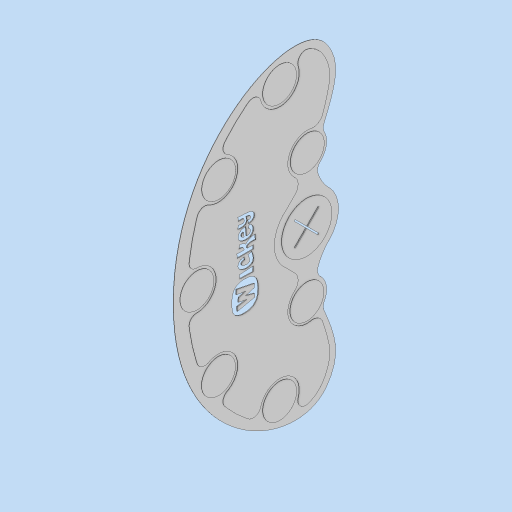
# Autodesk Inventor part: Sticker5
Saved by Autodesk Inventor 2024 (Build 280153000, 153)
## iProperties
Created: 2025-01-25
Part Number: Sticker5
Material: Generic
Document SubType Name: Modeling
Designer: Dmitry
Density: 1 g/cm^3
Appearance: Default
Author: Dmitry
Autodesk Inventor part; units mm, degrees
(part 1 of 2)
ref_plane "YZ Plane" through (0, 0, 0) normal (1, 0, 0) x (0, 1, 0)
ref_plane "XZ Plane" through (0, 0, 0) normal (0, 1, 0) x (-1, 0, 0)
ref_plane "XY Plane" through (0, 0, 0) normal (0, 0, 1) x (1, 0, 0)
sketch "Sketch1" plane through (0, 0, 0) normal (1, 0, 0) x (0, 1, 0)
  line L0 (189.6656, 2.8121) -> (188.0501, 2.8121)
  line L1 (188.0501, 2.8121) -> (183.2013, 3.4446)
  line L2 (183.2013, 3.4446) -> (176.455, 5.1464)
  line L3 (176.455, 5.1464) -> (169.3456, 7.6325)
  line L4 (169.3456, 7.6325) -> (163.6712, 9.8611)
  line L5 (163.6712, 9.8611) -> (161.7865, 10.6188)
  line L6 (161.7865, 10.6188) -> (160.3946, 11.1784)
  line L7 (160.3946, 11.1784) -> (156.2163, 12.8403)
  line L8 (137.2895, 19.2866) -> (130.161, 21.0285)
  line L9 (130.161, 21.0285) -> (122.5829, 22.3971)
  line L10 (108.1191, 23.6122) -> (105.9832, 23.6122)
  line L11 (105.9832, 23.6122) -> (105.6538, 23.6122)
  line L12 (103.6515, 23.6122) -> (103.3513, 23.6122)
  line L13 (103.3513, 23.6122) -> (101.2136, 23.6122)
  line L14 (86.7498, 22.3971) -> (79.1723, 21.0285)
  line L15 (79.1723, 21.0285) -> (72.0448, 19.2866)
  line L16 (48.9404, 11.1784) -> (47.5516, 10.6188)
  line L17 (47.5516, 10.6188) -> (45.6651, 9.8611)
  line L18 (45.6651, 9.8611) -> (39.9902, 7.6325)
  line L19 (39.9902, 7.6325) -> (32.8782, 5.1451)
  line L20 (32.8782, 5.1451) -> (26.1327, 3.4433)
  line L21 (26.1327, 3.4433) -> (21.2849, 2.8121)
  line L22 (21.2849, 2.8121) -> (19.67, 2.8121)
  line L23 (19.67, 2.8121) -> (18.5219, 2.8121)
  line L24 (18.5219, 2.8121) -> (15.0822, 3.1842)
  line L25 (15.0822, 3.1842) -> (10.6893, 4.3171)
  line L26 (10.6893, 4.3171) -> (6.4089, 6.2381)
  line L27 (6.4089, 6.2381) -> (3.179, 8.2239)
  line L28 (3.179, 8.2239) -> (2.1686, 8.9734)
  line L29 (2.1686, 8.9734) -> (1.3914, 9.551)
  line L30 (1.3914, 9.551) -> (-0.6922, 11.6137)
  line L31 (-0.6922, 11.6137) -> (-2.9411, 14.8096)
  line L32 (-2.9411, 14.8096) -> (-4.5728, 18.5121)
  line L33 (-4.5728, 18.5121) -> (-5.5802, 22.6739)
  line L34 (-5.5802, 22.6739) -> (-5.9535, 27.2477)
  line L35 (-5.9535, 27.2477) -> (-5.6861, 32.1824)
  line L36 (-5.6861, 32.1824) -> (-4.7712, 37.4326)
  line L37 (-4.7712, 37.4326) -> (-3.6589, 41.588)
  line L38 (-3.6589, 41.588) -> (-3.2004, 42.9444)
  line L39 (-3.2004, 42.9444) -> (-2.6889, 44.4633)
  line L40 (-2.6889, 44.4633) -> (-0.8492, 48.9159)
  line L41 (-0.8492, 48.9159) -> (2.1343, 54.8164)
  line L42 (2.1343, 54.8164) -> (5.7129, 60.5999)
  line L43 (5.7129, 60.5999) -> (9.8498, 66.221)
  line L44 (9.8498, 66.221) -> (14.5062, 71.6312)
  line L45 (14.5062, 71.6312) -> (19.6433, 76.7823)
  line L46 (19.6433, 76.7823) -> (25.2262, 81.6261)
  line L47 (25.2262, 81.6261) -> (29.6814, 85.05)
  line L48 (29.6814, 85.05) -> (31.2163, 86.1168)
  line L49 (31.2163, 86.1168) -> (33.089, 87.4198)
  line L50 (33.089, 87.4198) -> (38.929, 91.019)
  line L51 (38.929, 91.019) -> (47.0789, 95.2938)
  line L52 (47.0789, 95.2938) -> (55.631, 98.9387)
  line L53 (55.631, 98.9387) -> (64.5566, 101.9435)
  line L54 (64.5566, 101.9435) -> (73.8238, 104.2956)
  line L55 (73.8238, 104.2956) -> (83.3986, 105.9872)
  line L56 (83.3986, 105.9872) -> (93.2515, 107.0083)
  line L57 (93.2515, 107.0083) -> (100.825, 107.3512)
  line L58 (100.825, 107.3512) -> (103.3513, 107.3512)
  line L59 (103.3513, 107.3512) -> (103.6007, 107.3512)
  line L60 (103.6007, 107.3512) -> (104.2647, 107.3461)
  line L61 (104.2647, 107.3461) -> (104.3487, 107.3436)
  line L62 (104.3487, 107.3436) -> (104.6894, 107.341)
  line L63 (104.6894, 107.341) -> (104.9853, 107.3436)
  line L64 (104.9853, 107.3436) -> (105.0681, 107.3461)
  line L65 (105.0681, 107.3461) -> (105.7544, 107.3512)
  line L66 (105.7544, 107.3512) -> (105.9832, 107.3512)
  line L67 (105.9832, 107.3512) -> (108.5077, 107.3512)
  line L68 (108.5077, 107.3512) -> (116.0815, 107.0083)
  line L69 (116.0815, 107.0083) -> (125.9342, 105.9872)
  line L70 (125.9342, 105.9872) -> (135.509, 104.2956)
  line L71 (135.509, 104.2956) -> (144.7761, 101.9435)
  line L72 (144.7761, 101.9435) -> (153.7017, 98.9387)
  line L73 (153.7017, 98.9387) -> (162.2564, 95.2938)
  line L74 (162.2564, 95.2938) -> (170.4047, 91.019)
  line L75 (170.4047, 91.019) -> (176.2442, 87.4198)
  line L76 (176.2442, 87.4198) -> (178.1187, 86.1168)
  line L77 (178.1187, 86.1168) -> (179.6554, 85.05)
  line L78 (179.6554, 85.05) -> (184.108, 81.6261)
  line L79 (184.108, 81.6261) -> (189.691, 76.7823)
  line L80 (189.691, 76.7823) -> (194.8268, 71.6312)
  line L81 (194.8268, 71.6312) -> (199.4852, 66.221)
  line L82 (199.4852, 66.221) -> (203.6203, 60.5999)
  line L83 (203.6203, 60.5999) -> (207.1992, 54.8164)
  line L84 (207.1992, 54.8164) -> (210.1837, 48.9159)
  line L85 (210.1837, 48.9159) -> (212.0226, 44.4633)
  line L86 (212.0226, 44.4633) -> (212.5357, 42.9444)
  line L87 (212.5357, 42.9444) -> (212.9929, 41.588)
  line L88 (212.9929, 41.588) -> (214.1029, 37.4326)
  line L89 (214.1029, 37.4326) -> (215.0198, 32.1824)
  line L90 (215.0198, 32.1824) -> (215.2865, 27.2477)
  line L91 (215.2865, 27.2477) -> (214.9132, 22.6739)
  line L92 (214.9132, 22.6739) -> (213.9073, 18.5121)
  line L93 (213.9073, 18.5121) -> (212.2741, 14.8096)
  line L94 (212.2741, 14.8096) -> (210.0237, 11.6137)
  line L95 (210.0237, 11.6137) -> (207.9434, 9.5495)
  line L96 (207.9434, 9.5495) -> (207.1662, 8.9734)
  line L97 (207.1662, 8.9734) -> (206.1552, 8.2239)
  line L98 (206.1552, 8.2239) -> (202.9244, 6.2381)
  line L99 (202.9244, 6.2381) -> (198.647, 4.3171)
  line L100 (198.647, 4.3171) -> (194.2528, 3.1842)
  line L101 (194.2528, 3.1842) -> (190.8136, 2.8121)
  line L102 (190.8136, 2.8121) -> (189.6681, 2.8121)
  line L103 (189.6681, 2.8121) -> (189.6656, 2.8121)
  line L104 (205.0808, 10.3404) -> (204.0877, 9.6277)
  line L105 (204.0877, 9.6277) -> (200.9254, 7.7481)
  line L106 (200.9254, 7.7481) -> (196.7318, 5.928)
  line L107 (196.7318, 5.928) -> (192.4265, 4.8543)
  line L108 (192.4265, 4.8543) -> (189.0585, 4.5017)
  line L109 (189.0585, 4.5017) -> (187.9358, 4.5017)
  line L110 (187.9358, 4.5017) -> (186.8157, 4.5017)
  line L111 (186.8157, 4.5017) -> (183.4603, 4.9744)
  line L112 (183.4603, 4.9744) -> (178.0984, 6.1774)
  line L113 (178.0984, 6.1774) -> (172.4977, 7.7895)
  line L114 (172.4977, 7.7895) -> (168.5937, 9.045)
  line L115 (168.5937, 9.045) -> (167.3034, 9.4875)
  line L116 (167.3034, 9.4875) -> (166.7192, 9.6872)
  line L117 (166.7192, 9.6872) -> (165.1165, 10.7098)
  line L118 (165.1165, 10.7098) -> (163.5391, 12.5632)
  line L119 (163.5391, 12.5632) -> (162.7009, 14.8398)
  line L120 (162.7009, 14.8398) -> (162.6196, 16.7318)
  line L121 (162.6196, 16.7318) -> (162.7466, 17.3298)
  line L122 (162.7466, 17.3298) -> (162.8127, 17.6577)
  line L123 (162.8127, 17.6577) -> (163.0108, 19.3392)
  line L124 (163.0108, 19.3392) -> (163.0057, 21.074)
  line L125 (163.0057, 21.074) -> (162.9752, 21.4268)
  line L126 (162.9752, 21.4268) -> (162.9194, 22.0262)
  line L127 (162.9194, 22.0262) -> (162.5358, 23.804)
  line L128 (162.5358, 23.804) -> (161.7002, 26.0196)
  line L129 (161.7002, 26.0196) -> (160.5089, 28.0359)
  line L130 (160.5089, 28.0359) -> (159.0001, 29.8134)
  line L131 (159.0001, 29.8134) -> (157.2145, 31.3114)
  line L132 (157.2145, 31.3114) -> (155.1927, 32.4925)
  line L133 (155.1927, 32.4925) -> (152.9702, 33.315)
  line L134 (152.9702, 33.315) -> (151.1922, 33.6884)
  line L135 (151.1922, 33.6884) -> (150.5927, 33.7394)
  line L136 (150.5927, 33.7394) -> (149.7571, 33.8126)
  line L137 (149.7571, 33.8126) -> (147.2145, 33.6239)
  line L138 (147.2145, 33.6239) -> (144.0954, 32.7333)
  line L139 (144.0954, 32.7333) -> (141.3268, 31.1667)
  line L140 (141.3268, 31.1667) -> (139.5158, 29.6165)
  line L141 (139.5158, 29.6165) -> (139.0053, 29.0196)
  line L142 (139.0053, 29.0196) -> (138.5559, 28.4976)
  line L143 (138.5559, 28.4976) -> (136.7988, 27.2848)
  line L144 (136.7988, 27.2848) -> (134.2026, 26.5408)
  line L145 (134.2026, 26.5408) -> (131.5252, 26.8271)
  line L146 (131.5252, 26.8271) -> (129.5986, 27.7351)
  line L147 (129.5986, 27.7351) -> (129.0774, 28.1791)
  line L148 (129.0774, 28.1791) -> (128.4066, 28.7493)
  line L149 (128.4066, 28.7493) -> (122.1173, 34.9274)
  line L150 (122.1173, 34.9274) -> (121.5316, 35.5901)
  line L151 (121.5316, 35.5901) -> (121.4544, 35.6769)
  line L152 (121.4544, 35.6769) -> (120.655, 36.5284)
  line L153 (120.655, 36.5284) -> (120.5725, 36.6122)
  line L154 (120.5725, 36.6122) -> (119.7897, 37.392)
  line L155 (119.7897, 37.392) -> (117.1399, 39.4316)
  line L156 (117.1399, 39.4316) -> (113.2784, 41.4941)
  line L157 (113.2784, 41.4941) -> (109.0891, 42.759)
  line L158 (109.0891, 42.759) -> (105.7724, 43.1908)
  line L159 (105.7724, 43.1908) -> (104.667, 43.1908)
  line L160 (104.667, 43.1908) -> (103.5603, 43.1908)
  line L161 (103.5603, 43.1908) -> (100.2451, 42.759)
  line L162 (100.2451, 42.759) -> (96.0559, 41.4941)
  line L163 (96.0559, 41.4941) -> (92.1946, 39.4316)
  line L164 (92.1946, 39.4316) -> (89.5446, 37.392)
  line L165 (89.5446, 37.392) -> (88.7631, 36.6122)
  line L166 (88.7631, 36.6122) -> (88.6792, 36.5284)
  line L167 (88.6792, 36.5284) -> (87.8784, 35.6769)
  line L168 (87.8784, 35.6769) -> (87.8024, 35.5901)
  line L169 (87.8024, 35.5901) -> (87.2154, 34.9274)
  line L170 (87.2154, 34.9274) -> (80.9277, 28.7493)
  line L171 (80.9277, 28.7493) -> (80.2581, 28.1791)
  line L172 (80.2581, 28.1791) -> (79.7356, 27.7351)
  line L173 (79.7356, 27.7351) -> (77.809, 26.8271)
  line L174 (77.809, 26.8271) -> (75.1314, 26.5408)
  line L175 (75.1314, 26.5408) -> (72.5355, 27.2848)
  line L176 (72.5355, 27.2848) -> (70.7786, 28.4989)
  line L177 (70.7786, 28.4989) -> (70.3305, 29.0196)
  line L178 (70.3305, 29.0196) -> (69.818, 29.6165)
  line L179 (69.818, 29.6165) -> (68.0085, 31.1667)
  line L180 (68.0085, 31.1667) -> (65.2386, 32.7333)
  line L181 (65.2386, 32.7333) -> (62.1174, 33.6239)
  line L182 (62.1174, 33.6239) -> (59.5764, 33.8126)
  line L183 (59.5764, 33.8126) -> (58.7425, 33.7394)
  line L184 (58.7425, 33.7394) -> (58.1431, 33.6884)
  line L185 (58.1431, 33.6884) -> (56.3641, 33.315)
  line L186 (56.3641, 33.315) -> (54.1426, 32.4925)
  line L187 (54.1426, 32.4925) -> (52.1197, 31.3114)
  line L188 (52.1197, 31.3114) -> (50.3351, 29.8134)
  line L189 (50.3351, 29.8134) -> (48.8261, 28.0359)
  line L190 (48.8261, 28.0359) -> (47.6341, 26.0196)
  line L191 (47.6341, 26.0196) -> (46.7992, 23.804)
  line L192 (46.7992, 23.804) -> (46.4162, 22.0262)
  line L193 (46.4162, 22.0262) -> (46.3611, 21.4268)
  line L194 (46.3611, 21.4268) -> (46.3278, 21.074)
  line L195 (46.3278, 21.074) -> (46.3222, 19.3392)
  line L196 (46.3222, 19.3392) -> (46.5195, 17.6577)
  line L197 (46.5195, 17.6577) -> (46.5881, 17.3298)
  line L198 (46.5881, 17.3298) -> (46.7123, 16.7318)
  line L199 (46.7123, 16.7318) -> (46.6323, 14.8398)
  line L200 (46.6323, 14.8398) -> (45.7959, 12.5632)
  line L201 (45.7959, 12.5632) -> (44.2183, 10.7098)
  line L202 (44.2183, 10.7098) -> (42.614, 9.6872)
  line L203 (42.614, 9.6872) -> (42.0324, 9.4875)
  line L204 (42.0324, 9.4875) -> (40.7398, 9.045)
  line L205 (40.7398, 9.045) -> (36.8373, 7.7895)
  line L206 (36.8373, 7.7895) -> (31.2343, 6.1774)
  line L207 (31.2343, 6.1774) -> (25.8724, 4.9744)
  line L208 (25.8724, 4.9744) -> (22.5181, 4.5017)
  line L209 (22.5181, 4.5017) -> (21.4005, 4.5017)
  line L210 (21.4005, 4.5017) -> (20.276, 4.5017)
  line L211 (20.276, 4.5017) -> (16.907, 4.8543)
  line L212 (16.907, 4.8543) -> (12.6017, 5.928)
  line L213 (12.6017, 5.928) -> (8.4099, 7.7481)
  line L214 (8.4099, 7.7481) -> (5.2473, 9.6277)
  line L215 (5.2473, 9.6277) -> (4.255, 10.3404)
  line L216 (4.255, 10.3404) -> (3.4777, 10.8985)
  line L217 (3.4777, 10.8985) -> (0.2644, 14.312)
  line L218 (0.2644, 14.312) -> (-2.0397, 18.4847)
  line L219 (-2.0397, 18.4847) -> (-2.3625, 19.423)
  line L220 (-2.3625, 19.423) -> (-2.4933, 19.8047)
  line L221 (-2.4933, 19.8047) -> (-2.6683, 21.0244)
  line L222 (-2.6683, 21.0244) -> (-2.5085, 22.5403)
  line L223 (-2.5085, 22.5403) -> (-1.9477, 23.9101)
  line L224 (-1.9477, 23.9101) -> (-1.0506, 25.0704)
  line L225 (-1.0506, 25.0704) -> (0.1196, 25.9604)
  line L226 (0.1196, 25.9604) -> (1.4991, 26.5172)
  line L227 (1.4991, 26.5172) -> (3.0243, 26.6782)
  line L228 (3.0243, 26.6782) -> (4.2481, 26.5119)
  line L229 (4.2481, 26.5119) -> (4.6327, 26.3833)
  line L230 (4.6327, 26.3833) -> (4.6408, 26.3808)
  line L231 (4.6408, 26.3808) -> (4.7332, 26.3506)
  line L232 (4.7332, 26.3506) -> (4.7429, 26.3463)
  line L233 (4.7429, 26.3463) -> (5.4236, 26.1258)
  line L234 (5.4236, 26.1258) -> (7.5623, 25.7499)
  line L235 (7.5623, 25.7499) -> (10.3596, 25.7499)
  line L236 (10.3596, 25.7499) -> (13.0553, 26.3104)
  line L237 (13.0553, 26.3104) -> (15.5702, 27.3882)
  line L238 (15.5702, 27.3882) -> (17.8244, 28.9452)
  line L239 (17.8244, 28.9452) -> (19.7401, 30.9396)
  line L240 (19.7401, 30.9396) -> (21.2351, 33.3302)
  line L241 (21.2351, 33.3302) -> (22.0593, 35.3724)
  line L242 (22.0593, 35.3724) -> (22.2341, 36.0762)
  line L243 (22.2341, 36.0762) -> (22.3832, 36.6833)
  line L244 (22.3832, 36.6833) -> (22.6077, 38.5553)
  line L245 (22.6077, 38.5553) -> (22.5234, 41.0038)
  line L246 (22.5234, 41.0038) -> (22.0096, 43.3711)
  line L247 (22.0096, 43.3711) -> (21.0934, 45.6038)
  line L248 (21.0934, 45.6038) -> (19.8046, 47.6409)
  line L249 (19.8046, 47.6409) -> (18.1719, 49.4316)
  line L250 (18.1719, 49.4316) -> (16.2247, 50.92)
  line L251 (16.2247, 50.92) -> (14.5684, 51.8217)
  line L252 (14.5684, 51.8217) -> (13.9895, 52.0503)
  line L253 (13.9895, 52.0503) -> (13.8419, 52.1062)
  line L254 (13.8419, 52.1062) -> (12.3634, 52.5786)
  line L255 (12.3634, 52.5786) -> (12.2161, 52.6142)
  line L256 (12.2161, 52.6142) -> (11.8755, 52.698)
  line L257 (11.8755, 52.698) -> (10.8983, 53.1222)
  line L258 (10.8983, 53.1222) -> (9.8059, 53.9045)
  line L259 (9.8059, 53.9045) -> (8.9557, 54.9078)
  line L260 (8.9557, 54.9078) -> (8.3698, 56.0711)
  line L261 (8.3698, 56.0711) -> (8.0723, 57.336)
  line L262 (8.0723, 57.336) -> (8.0817, 58.6467)
  line L263 (8.0817, 58.6467) -> (8.4195, 59.9472)
  line L264 (8.4195, 59.9472) -> (8.9016, 60.8946)
  line L265 (8.9016, 60.8946) -> (9.1099, 61.174)
  line L266 (9.1099, 61.174) -> (10.2067, 62.6548)
  line L267 (10.2067, 62.6548) -> (16.3967, 69.7744)
  line L268 (16.3967, 69.7744) -> (23.4495, 76.447)
  line L269 (23.4495, 76.447) -> (24.9791, 77.6992)
  line L270 (24.9791, 77.6992) -> (25.4353, 78.0751)
  line L271 (25.4353, 78.0751) -> (27.1579, 78.7711)
  line L272 (27.1579, 78.7711) -> (29.4772, 78.7711)
  line L273 (29.4772, 78.7711) -> (31.5981, 77.7881)
  line L274 (31.5981, 77.7881) -> (32.9016, 76.447)
  line L275 (32.9016, 76.447) -> (33.1787, 75.9161)
  line L276 (33.1787, 75.9161) -> (33.1993, 75.8755)
  line L277 (33.1993, 75.8755) -> (33.4269, 75.4615)
  line L278 (33.4269, 75.4615) -> (33.4515, 75.4208)
  line L279 (33.4515, 75.4208) -> (33.8084, 74.8011)
  line L280 (33.8084, 74.8011) -> (35.1464, 73.0917)
  line L281 (35.1464, 73.0917) -> (37.2259, 71.2197)
  line L282 (37.2259, 71.2197) -> (39.6044, 69.8328)
  line L283 (39.6044, 69.8328) -> (42.1952, 68.9489)
  line L284 (42.1952, 68.9489) -> (44.9112, 68.5984)
  line L285 (44.9112, 68.5984) -> (47.6686, 68.7991)
  line L286 (47.6686, 68.7991) -> (50.3806, 69.5763)
  line L287 (50.3806, 69.5763) -> (52.3598, 70.5415)
  line L288 (52.3598, 70.5415) -> (52.9618, 70.9504)
  line L289 (52.9618, 70.9504) -> (53.4675, 71.2933)
  line L290 (53.4675, 71.2933) -> (54.8609, 72.5049)
  line L291 (54.8609, 72.5049) -> (56.4167, 74.3363)
  line L292 (56.4167, 74.3363) -> (57.6153, 76.386)
  line L293 (57.6153, 76.386) -> (58.4408, 78.6035)
  line L294 (58.4408, 78.6035) -> (58.8761, 80.9276)
  line L295 (58.8761, 80.9276) -> (58.9066, 83.305)
  line L296 (58.9066, 83.305) -> (58.5167, 85.6748)
  line L297 (58.5167, 85.6748) -> (57.9462, 87.4325)
  line L298 (57.9462, 87.4325) -> (57.6897, 87.9837)
  line L299 (57.6897, 87.9837) -> (57.6486, 88.0726)
  line L300 (57.6486, 88.0726) -> (57.2157, 88.9133)
  line L301 (57.2157, 88.9133) -> (57.17, 88.9946)
  line L302 (57.17, 88.9946) -> (56.8779, 89.5102)
  line L303 (56.8779, 89.5102) -> (56.4621, 91.3136)
  line L304 (56.4621, 91.3136) -> (56.7845, 93.6047)
  line L305 (56.7845, 93.6047) -> (58.026, 95.5453)
  line L306 (58.026, 95.5453) -> (59.5226, 96.6171)
  line L307 (59.5226, 96.6171) -> (60.0791, 96.8026)
  line L308 (60.0791, 96.8026) -> (62.0829, 97.4731)
  line L309 (62.0829, 97.4731) -> (72.4278, 100.229)
  line L310 (72.4278, 100.229) -> (83.1657, 102.195)
  line L311 (83.1657, 102.195) -> (85.3676, 102.4668)
  line L312 (85.3676, 102.4668) -> (85.6416, 102.4998)
  line L313 (85.6416, 102.4998) -> (86.4796, 102.482)
  line L314 (86.4796, 102.482) -> (87.5271, 102.2636)
  line L315 (87.5271, 102.2636) -> (88.4849, 101.8368)
  line L316 (88.4849, 101.8368) -> (89.3269, 101.2247)
  line L317 (89.3269, 101.2247) -> (90.0239, 100.45)
  line L318 (90.0239, 100.45) -> (90.5545, 99.5407)
  line L319 (90.5545, 99.5407) -> (90.8893, 98.5171)
  line L320 (90.8893, 98.5171) -> (91.0041, 97.6839)
  line L321 (91.0041, 97.6839) -> (91.0041, 97.4071)
  line L322 (91.0041, 97.4071) -> (91.0041, 97.3918)
  line L323 (91.0041, 97.3918) -> (91.0041, 97.3563)
  line L324 (91.0041, 97.3563) -> (91.0041, 97.3436)
  line L325 (91.0041, 97.3436) -> (91.0041, 96.6578)
  line L326 (91.0041, 96.6578) -> (91.281, 94.5953)
  line L327 (91.281, 94.5953) -> (92.079, 92.0324)
  line L328 (92.079, 92.0324) -> (93.3396, 89.7134)
  line L329 (93.3396, 89.7134) -> (95.0097, 87.689)
  line L330 (95.0097, 87.689) -> (97.0325, 86.0203)
  line L331 (97.0325, 86.0203) -> (99.3536, 84.7604)
  line L332 (99.3536, 84.7604) -> (101.9164, 83.9629)
  line L333 (101.9164, 83.9629) -> (103.9794, 83.686)
  line L334 (103.9794, 83.686) -> (104.667, 83.686)
  line L335 (104.667, 83.686) -> (105.3533, 83.686)
  line L336 (105.3533, 83.686) -> (107.4163, 83.9629)
  line L337 (107.4163, 83.9629) -> (109.9797, 84.7604)
  line L338 (109.9797, 84.7604) -> (112.3002, 86.0203)
  line L339 (112.3002, 86.0203) -> (114.3243, 87.689)
  line L340 (114.3243, 87.689) -> (115.9944, 89.7134)
  line L341 (115.9944, 89.7134) -> (117.2555, 92.0324)
  line L342 (117.2555, 92.0324) -> (118.0533, 94.5953)
  line L343 (118.0533, 94.5953) -> (118.3314, 96.6578)
  line L344 (118.3314, 96.6578) -> (118.3314, 97.3436)
  line L345 (118.3314, 97.3436) -> (118.3314, 97.3614)
  line L346 (118.3314, 97.3614) -> (118.3304, 97.402)
  line L347 (118.3304, 97.402) -> (118.3304, 97.4071)
  line L348 (118.3304, 97.4071) -> (118.3292, 97.6839)
  line L349 (118.3292, 97.6839) -> (118.4435, 98.5171)
  line L350 (118.4435, 98.5171) -> (118.7782, 99.5407)
  line L351 (118.7782, 99.5407) -> (119.3088, 100.45)
  line L352 (119.3088, 100.45) -> (120.0073, 101.2247)
  line L353 (120.0073, 101.2247) -> (120.8478, 101.8368)
  line L354 (120.8478, 101.8368) -> (121.8057, 102.2636)
  line L355 (121.8057, 102.2636) -> (122.8544, 102.482)
  line L356 (122.8544, 102.482) -> (123.6924, 102.4998)
  line L357 (123.6924, 102.4998) -> (123.968, 102.4668)
  line L358 (123.968, 102.4668) -> (126.1686, 102.195)
  line L359 (126.1686, 102.195) -> (136.9077, 100.229)
  line L360 (136.9077, 100.229) -> (147.2501, 97.4731)
  line L361 (147.2501, 97.4731) -> (149.2567, 96.8026)
  line L362 (149.2567, 96.8026) -> (149.813, 96.6171)
  line L363 (149.813, 96.6171) -> (151.309, 95.5453)
  line L364 (151.309, 95.5453) -> (152.5511, 93.6047)
  line L365 (152.5511, 93.6047) -> (152.8711, 91.3136)
  line L366 (152.8711, 91.3136) -> (152.4546, 89.5077)
  line L367 (152.4546, 89.5077) -> (152.165, 88.9946)
  line L368 (152.165, 88.9946) -> (152.1167, 88.9133)
  line L369 (152.1167, 88.9133) -> (151.6849, 88.0726)
  line L370 (151.6849, 88.0726) -> (151.6443, 87.9837)
  line L371 (151.6443, 87.9837) -> (151.3878, 87.4325)
  line L372 (151.3878, 87.4325) -> (150.8163, 85.6748)
  line L373 (150.8163, 85.6748) -> (150.4251, 83.305)
  line L374 (150.4251, 83.305) -> (150.4556, 80.9276)
  line L375 (150.4556, 80.9276) -> (150.8925, 78.6035)
  line L376 (150.8925, 78.6035) -> (151.718, 76.386)
  line L377 (151.718, 76.386) -> (152.9168, 74.3363)
  line L378 (152.9168, 74.3363) -> (154.4739, 72.5049)
  line L379 (154.4739, 72.5049) -> (155.8658, 71.2933)
  line L380 (155.8658, 71.2933) -> (156.3738, 70.9504)
  line L381 (156.3738, 70.9504) -> (156.9732, 70.5415)
  line L382 (156.9732, 70.5415) -> (158.9519, 69.5763)
  line L383 (158.9519, 69.5763) -> (161.6646, 68.7991)
  line L384 (161.6646, 68.7991) -> (164.4205, 68.5984)
  line L385 (164.4205, 68.5984) -> (167.1383, 68.9489)
  line L386 (167.1383, 68.9489) -> (169.7291, 69.8328)
  line L387 (169.7291, 69.8328) -> (172.1091, 71.2197)
  line L388 (172.1091, 71.2197) -> (174.1868, 73.0917)
  line L389 (174.1868, 73.0917) -> (175.5254, 74.8011)
  line L390 (175.5254, 74.8011) -> (175.8835, 75.4208)
  line L391 (175.8835, 75.4208) -> (175.9089, 75.4615)
  line L392 (175.9089, 75.4615) -> (176.1324, 75.8755)
  line L393 (176.1324, 75.8755) -> (176.1553, 75.9161)
  line L394 (176.1553, 75.9161) -> (176.4322, 76.447)
  line L395 (176.4322, 76.447) -> (177.7352, 77.7881)
  line L396 (177.7352, 77.7881) -> (179.8561, 78.7711)
  line L397 (179.8561, 78.7711) -> (182.1751, 78.7711)
  line L398 (182.1751, 78.7711) -> (183.8998, 78.0751)
  line L399 (183.8998, 78.0751) -> (184.357, 77.6992)
  line L400 (184.357, 77.6992) -> (185.8835, 76.447)
  line L401 (185.8835, 76.447) -> (192.9371, 69.7744)
  line L402 (192.9371, 69.7744) -> (199.1271, 62.6548)
  line L403 (199.1271, 62.6548) -> (200.2269, 61.174)
  line L404 (200.2269, 61.174) -> (200.4352, 60.8946)
  line L405 (200.4352, 60.8946) -> (200.9152, 59.9472)
  line L406 (200.9152, 59.9472) -> (201.253, 58.6467)
  line L407 (201.253, 58.6467) -> (201.2632, 57.336)
  line L408 (201.2632, 57.336) -> (200.9635, 56.0711)
  line L409 (200.9635, 56.0711) -> (200.3767, 54.9078)
  line L410 (200.3767, 54.9078) -> (199.5284, 53.9045)
  line L411 (199.5284, 53.9045) -> (198.4336, 53.1222)
  line L412 (198.4336, 53.1222) -> (197.4583, 52.698)
  line L413 (197.4583, 52.698) -> (197.1179, 52.6142)
  line L414 (197.1179, 52.6142) -> (196.9706, 52.5786)
  line L415 (196.9706, 52.5786) -> (195.4923, 52.1062)
  line L416 (195.4923, 52.1062) -> (195.345, 52.0503)
  line L417 (195.345, 52.0503) -> (194.7659, 51.8217)
  line L418 (194.7659, 51.8217) -> (193.1098, 50.92)
  line L419 (193.1098, 50.92) -> (191.1616, 49.4316)
  line L420 (191.1616, 49.4316) -> (189.5284, 47.6409)
  line L421 (189.5284, 47.6409) -> (188.2406, 45.6038)
  line L422 (188.2406, 45.6038) -> (187.3237, 43.3711)
  line L423 (187.3237, 43.3711) -> (186.8106, 41.0038)
  line L424 (186.8106, 41.0038) -> (186.7268, 38.5553)
  line L425 (186.7268, 38.5553) -> (186.9503, 36.6833)
  line L426 (186.9503, 36.6833) -> (187.1002, 36.0762)
  line L427 (187.1002, 36.0762) -> (187.2754, 35.3724)
  line L428 (187.2754, 35.3724) -> (188.0984, 33.3302)
  line L429 (188.0984, 33.3302) -> (189.5944, 30.9396)
  line L430 (189.5944, 30.9396) -> (191.5096, 28.9452)
  line L431 (191.5096, 28.9452) -> (193.7651, 27.3882)
  line L432 (193.7651, 27.3882) -> (196.2797, 26.3104)
  line L433 (196.2797, 26.3104) -> (198.9747, 25.7499)
  line L434 (198.9747, 25.7499) -> (201.7712, 25.7499)
  line L435 (201.7712, 25.7499) -> (203.9099, 26.1258)
  line L436 (203.9099, 26.1258) -> (204.5931, 26.3463)
  line L437 (204.5931, 26.3463) -> (204.6008, 26.3506)
  line L438 (204.6008, 26.3506) -> (204.6922, 26.3808)
  line L439 (204.6922, 26.3808) -> (204.7024, 26.3833)
  line L440 (204.7024, 26.3833) -> (205.0859, 26.5119)
  line L441 (205.0859, 26.5119) -> (206.3076, 26.6782)
  line L442 (206.3076, 26.6782) -> (207.8342, 26.5172)
  line L443 (207.8342, 26.5172) -> (209.2134, 25.9604)
  line L444 (209.2134, 25.9604) -> (210.3843, 25.0704)
  line L445 (210.3843, 25.0704) -> (211.281, 23.9101)
  line L446 (211.281, 23.9101) -> (211.8423, 22.5403)
  line L447 (211.8423, 22.5403) -> (212.0023, 21.0244)
  line L448 (212.0023, 21.0244) -> (211.8271, 19.8047)
  line L449 (211.8271, 19.8047) -> (211.6975, 19.423)
  line L450 (211.6975, 19.423) -> (211.3749, 18.4847)
  line L451 (211.3749, 18.4847) -> (209.0686, 14.312)
  line L452 (209.0686, 14.312) -> (205.8581, 10.8985)
  line L453 (205.8581, 10.8985) -> (205.0808, 10.3404)
  line L454 (105.9843, 113.216) -> (105.6553, 113.216)
  line L455 (105.6553, 113.216) -> (104.776, 113.2084)
  line L456 (104.776, 113.2084) -> (104.667, 113.2059)
  line L457 (104.667, 113.2059) -> (104.557, 113.2084)
  line L458 (104.557, 113.2084) -> (103.6515, 113.216)
  line L459 (103.6515, 113.216) -> (103.3513, 113.216)
  line L460 (103.3513, 113.216) -> (101.2207, 113.216)
  line L461 (101.2207, 113.216) -> (94.8334, 112.9747)
  line L462 (94.8334, 112.9747) -> (86.6355, 112.261)
  line L463 (86.6355, 112.261) -> (78.7615, 111.1078)
  line L464 (78.7615, 111.1078) -> (71.2111, 109.5381)
  line L465 (71.2111, 109.5381) -> (63.9876, 107.5823)
  line L466 (63.9876, 107.5823) -> (57.0933, 105.2658)
  line L467 (57.0933, 105.2658) -> (50.531, 102.6141)
  line L468 (50.531, 102.6141) -> (44.3009, 99.6575)
  line L469 (44.3009, 99.6575) -> (38.407, 96.4216)
  line L470 (38.407, 96.4216) -> (32.8508, 92.9341)
  line L471 (32.8508, 92.9341) -> (27.6349, 89.2181)
  line L472 (27.6349, 89.2181) -> (22.7619, 85.304)
  line L473 (22.7619, 85.304) -> (18.2323, 81.2197)
  line L474 (18.2323, 81.2197) -> (14.0515, 76.9906)
  line L475 (14.0515, 76.9906) -> (10.2194, 72.6446)
  line L476 (10.2194, 72.6446) -> (6.7381, 68.2072)
  line L477 (6.7381, 68.2072) -> (3.6101, 63.7089)
  line L478 (3.6101, 63.7089) -> (0.8389, 59.1725)
  line L479 (0.8389, 59.1725) -> (-1.5754, 54.6284)
  line L480 (-1.5754, 54.6284) -> (-3.6287, 50.1021)
  line L481 (-3.6287, 50.1021) -> (-5.3196, 45.619)
  line L482 (-5.3196, 45.619) -> (-6.6452, 41.207)
  line L483 (-6.6452, 41.207) -> (-7.6045, 36.8941)
  line L484 (-7.6045, 36.8941) -> (-8.1943, 32.71)
  line L485 (-8.1943, 32.71) -> (-8.412, 28.6764)
  line L486 (-8.412, 28.6764) -> (-8.2573, 24.8248)
  line L487 (-8.2573, 24.8248) -> (-7.7257, 21.1789)
  line L488 (-7.7257, 21.1789) -> (-6.8164, 17.7669)
  line L489 (-6.8164, 17.7669) -> (-5.5263, 14.6165)
  line L490 (-5.5263, 14.6165) -> (-3.8535, 11.7545)
  line L491 (-3.8535, 11.7545) -> (-1.7961, 9.2076)
  line L492 (-1.7961, 9.2076) -> (-0.0018, 7.5017)
  line L493 (-0.0018, 7.5017) -> (0.6502, 7.0014)
  line L494 (0.6502, 7.0014) -> (2.0045, 5.9625)
  line L495 (2.0045, 5.9625) -> (6.4335, 3.3153)
  line L496 (6.4335, 3.3153) -> (12.1346, 1.1075)
  line L497 (12.1346, 1.1075) -> (17.8191, 0.1886)
  line L498 (17.8191, 0.1886) -> (23.5544, 0.3717)
  line L499 (23.5544, 0.3717) -> (29.4096, 1.4697)
  line L500 (29.4096, 1.4697) -> (35.4538, 3.2945)
  line L501 (35.4538, 3.2945) -> (41.7527, 5.659)
  line L502 (41.7527, 5.659) -> (46.7233, 7.6889)
  line L503 (46.7233, 7.6889) -> (48.3771, 8.3755)
  line L504 (48.3771, 8.3755) -> (48.676, 8.5007)
  line L505 (48.676, 8.5007) -> (49.6295, 8.7446)
  line L506 (49.6295, 8.7446) -> (50.9183, 8.834)
  line L507 (50.9183, 8.834) -> (52.1914, 8.6371)
  line L508 (52.1914, 8.6371) -> (53.1147, 8.3036)
  line L509 (53.1147, 8.3036) -> (53.3986, 8.1479)
  line L510 (53.3986, 8.1479) -> (53.885, 7.8805)
  line L511 (53.885, 7.8805) -> (56.52, 6.9051)
  line L512 (56.52, 6.9051) -> (59.1022, 6.4654)
  line L513 (59.1022, 6.4654) -> (59.9635, 6.4654)
  line L514 (59.9635, 6.4654) -> (60.6925, 6.4654)
  line L515 (60.6925, 6.4654) -> (62.881, 6.7796)
  line L516 (62.881, 6.7796) -> (65.5817, 7.6767)
  line L517 (65.5817, 7.6767) -> (68.0019, 9.0892)
  line L518 (68.0019, 9.0892) -> (69.6084, 10.4382)
  line L519 (69.6084, 10.4382) -> (70.0745, 10.9508)
  line L520 (70.0745, 10.9508) -> (70.3458, 11.2513)
  line L521 (70.3458, 11.2513) -> (71.3404, 11.9902)
  line L522 (71.3404, 11.9902) -> (72.8246, 12.6155)
  line L523 (72.8246, 12.6155) -> (74.4273, 12.8086)
  line L524 (74.4273, 12.8086) -> (75.662, 12.6706)
  line L525 (75.662, 12.6706) -> (76.0521, 12.552)
  line L526 (76.0521, 12.552) -> (76.9256, 12.2874)
  line L527 (76.9256, 12.2874) -> (79.4847, 11.2731)
  line L528 (79.4847, 11.2731) -> (82.7549, 9.5673)
  line L529 (82.7549, 9.5673) -> (85.821, 7.4481)
  line L530 (85.821, 7.4481) -> (87.9779, 5.596)
  line L531 (87.9779, 5.596) -> (88.6404, 4.9231)
  line L532 (88.6404, 4.9231) -> (88.6503, 4.9137)
  line L533 (88.6503, 4.9137) -> (88.7521, 4.8116)
  line L534 (88.7521, 4.8116) -> (88.7631, 4.8007)
  line L535 (88.7631, 4.8007) -> (89.5446, 4.0194)
  line L536 (89.5446, 4.0194) -> (92.1946, 1.98)
  line L537 (92.1946, 1.98) -> (96.0559, -0.0845)
  line L538 (96.0559, -0.0845) -> (100.2451, -1.3509)
  line L539 (100.2451, -1.3509) -> (103.5603, -1.7835)
  line L540 (103.5603, -1.7835) -> (104.667, -1.7835)
  line L541 (104.667, -1.7835) -> (105.7724, -1.7835)
  line L542 (105.7724, -1.7835) -> (109.0891, -1.3509)
  line L543 (109.0891, -1.3509) -> (113.2784, -0.0845)
  line L544 (113.2784, -0.0845) -> (117.1399, 1.98)
  line L545 (117.1399, 1.98) -> (119.7897, 4.0194)
  line L546 (119.7897, 4.0194) -> (120.5725, 4.8007)
  line L547 (120.5725, 4.8007) -> (120.5819, 4.8116)
  line L548 (120.5819, 4.8116) -> (120.684, 4.9137)
  line L549 (120.684, 4.9137) -> (120.6952, 4.9231)
  line L550 (120.6952, 4.9231) -> (121.3566, 5.596)
  line L551 (121.3566, 5.596) -> (123.5133, 7.4481)
  line L552 (123.5133, 7.4481) -> (126.5778, 9.5673)
  line L553 (126.5778, 9.5673) -> (129.8481, 11.2731)
  line L554 (129.8481, 11.2731) -> (132.4071, 12.2863)
  line L555 (132.4071, 12.2863) -> (133.2819, 12.552)
  line L556 (133.2819, 12.552) -> (133.6708, 12.6706)
  line L557 (133.6708, 12.6706) -> (134.9055, 12.8086)
  line L558 (134.9055, 12.8086) -> (136.5095, 12.6155)
  line L559 (136.5095, 12.6155) -> (137.9936, 11.9902)
  line L560 (137.9936, 11.9902) -> (138.9875, 11.2513)
  line L561 (138.9875, 11.2513) -> (139.2618, 10.9508)
  line L562 (139.2618, 10.9508) -> (139.7266, 10.4382)
  line L563 (139.7266, 10.4382) -> (141.3319, 9.0892)
  line L564 (141.3319, 9.0892) -> (143.75, 7.6767)
  line L565 (143.75, 7.6767) -> (146.4525, 6.7796)
  line L566 (146.4525, 6.7796) -> (148.6395, 6.4654)
  line L567 (148.6395, 6.4654) -> (149.371, 6.4654)
  line L568 (149.371, 6.4654) -> (150.2295, 6.4654)
  line L569 (150.2295, 6.4654) -> (152.8152, 6.9051)
  line L570 (152.8152, 6.9051) -> (155.4467, 7.8805)
  line L571 (155.4467, 7.8805) -> (155.9344, 8.1479)
  line L572 (155.9344, 8.1479) -> (156.2188, 8.3036)
  line L573 (156.2188, 8.3036) -> (157.1409, 8.6371)
  line L574 (157.1409, 8.6371) -> (158.4159, 8.834)
  line L575 (158.4159, 8.834) -> (159.7037, 8.7446)
  line L576 (159.7037, 8.7446) -> (160.6588, 8.5007)
  line L577 (160.6588, 8.5007) -> (160.9585, 8.3755)
  line L578 (160.9585, 8.3755) -> (162.6095, 7.6889)
  line L579 (162.6095, 7.6889) -> (167.5803, 5.659)
  line L580 (167.5803, 5.659) -> (173.8795, 3.2945)
  line L581 (173.8795, 3.2945) -> (179.9221, 1.4697)
  line L582 (179.9221, 1.4697) -> (185.7794, 0.3717)
  line L583 (185.7794, 0.3717) -> (191.5147, 0.1886)
  line L584 (191.5147, 0.1886) -> (197.1992, 1.1075)
  line L585 (197.1992, 1.1075) -> (202.899, 3.3153)
  line L586 (202.899, 3.3153) -> (207.3287, 5.9625)
  line L587 (207.3287, 5.9625) -> (208.6851, 7.0014)
  line L588 (208.6851, 7.0014) -> (209.3353, 7.5017)
  line L589 (209.3353, 7.5017) -> (211.1286, 9.2076)
  line L590 (211.1286, 9.2076) -> (213.186, 11.7545)
  line L591 (213.186, 11.7545) -> (214.8598, 14.6165)
  line L592 (214.8598, 14.6165) -> (216.1501, 17.7669)
  line L593 (216.1501, 17.7669) -> (217.0595, 21.1789)
  line L594 (217.0595, 21.1789) -> (217.5903, 24.8248)
  line L595 (217.5903, 24.8248) -> (217.7453, 28.6764)
  line L596 (217.7453, 28.6764) -> (217.5294, 32.71)
  line L597 (217.5294, 32.71) -> (216.9375, 36.8941)
  line L598 (216.9375, 36.8941) -> (215.98, 41.207)
  line L599 (215.98, 41.207) -> (214.6541, 45.619)
  line L600 (214.6541, 45.619) -> (212.9624, 50.1021)
  line L601 (212.9624, 50.1021) -> (210.9101, 54.6284)
  line L602 (210.9101, 54.6284) -> (208.4946, 59.1725)
  line L603 (208.4946, 59.1725) -> (205.7234, 63.7089)
  line L604 (205.7234, 63.7089) -> (202.5967, 68.2072)
  line L605 (202.5967, 68.2072) -> (199.1144, 72.6446)
  line L606 (199.1144, 72.6446) -> (195.2815, 76.9906)
  line L607 (195.2815, 76.9906) -> (191.1007, 81.2197)
  line L608 (191.1007, 81.2197) -> (186.5718, 85.304)
  line L609 (186.5718, 85.304) -> (181.7001, 89.2181)
  line L610 (181.7001, 89.2181) -> (176.483, 92.9341)
  line L611 (176.483, 92.9341) -> (170.928, 96.4216)
  line L612 (170.928, 96.4216) -> (165.0326, 99.6575)
  line L613 (165.0326, 99.6575) -> (158.8046, 102.6141)
  line L614 (158.8046, 102.6141) -> (152.2412, 105.2658)
  line L615 (152.2412, 105.2658) -> (145.3476, 107.5823)
  line L616 (145.3476, 107.5823) -> (138.1231, 109.5381)
  line L617 (138.1231, 109.5381) -> (130.573, 111.1078)
  line L618 (130.573, 111.1078) -> (122.6987, 112.261)
  line L619 (122.6987, 112.261) -> (114.5009, 112.9747)
  line L620 (114.5009, 112.9747) -> (108.1138, 113.216)
  line L621 (108.1138, 113.216) -> (105.9843, 113.216)
  line L622 (161.149, 20.1286) -> (161.149, 19.536)
  line L623 (161.149, 19.536) -> (160.9102, 17.7555)
  line L624 (160.9102, 17.7555) -> (160.2244, 15.5439)
  line L625 (160.2244, 15.5439) -> (159.1373, 13.5429)
  line L626 (159.1373, 13.5429) -> (157.6997, 11.7999)
  line L627 (157.6997, 11.7999) -> (155.9572, 10.361)
  line L628 (155.9572, 10.361) -> (153.9557, 9.2752)
  line L629 (153.9557, 9.2752) -> (151.7434, 8.5889)
  line L630 (151.7434, 8.5889) -> (149.9628, 8.3491)
  line L631 (149.9628, 8.3491) -> (149.371, 8.3491)
  line L632 (149.371, 8.3491) -> (148.7766, 8.3491)
  line L633 (148.7766, 8.3491) -> (146.9961, 8.5889)
  line L634 (146.9961, 8.5889) -> (144.7863, 9.2752)
  line L635 (144.7863, 9.2752) -> (142.7848, 10.361)
  line L636 (142.7848, 10.361) -> (141.0423, 11.7999)
  line L637 (141.0423, 11.7999) -> (139.6022, 13.5429)
  line L638 (139.6022, 13.5429) -> (138.5171, 15.5439)
  line L639 (138.5171, 15.5439) -> (137.831, 17.7555)
  line L640 (137.831, 17.7555) -> (137.5925, 19.536)
  line L641 (137.5925, 19.536) -> (137.5925, 20.1286)
  line L642 (137.5925, 20.1286) -> (137.5925, 20.7227)
  line L643 (137.5925, 20.7227) -> (137.831, 22.5027)
  line L644 (137.831, 22.5027) -> (138.5171, 24.7148)
  line L645 (138.5171, 24.7148) -> (139.6022, 26.7158)
  line L646 (139.6022, 26.7158) -> (141.0423, 28.4588)
  line L647 (141.0423, 28.4588) -> (142.7848, 29.8974)
  line L648 (142.7848, 29.8974) -> (144.7863, 30.9835)
  line L649 (144.7863, 30.9835) -> (146.9961, 31.6698)
  line L650 (146.9961, 31.6698) -> (148.7766, 31.9083)
  line L651 (148.7766, 31.9083) -> (149.371, 31.9083)
  line L652 (149.371, 31.9083) -> (149.9628, 31.9083)
  line L653 (149.9628, 31.9083) -> (151.7434, 31.6698)
  line L654 (151.7434, 31.6698) -> (153.9557, 30.9835)
  line L655 (153.9557, 30.9835) -> (155.9572, 29.8974)
  line L656 (155.9572, 29.8974) -> (157.6997, 28.4588)
  line L657 (157.6997, 28.4588) -> (159.1373, 26.7158)
  line L658 (159.1373, 26.7158) -> (160.2244, 24.7148)
  line L659 (160.2244, 24.7148) -> (160.9102, 22.5027)
  line L660 (160.9102, 22.5027) -> (161.149, 20.7227)
  line L661 (161.149, 20.7227) -> (161.149, 20.1286)
  line L662 (47.8396, 20.3861) -> (47.8396, 19.7938)
  line L663 (47.8396, 19.7938) -> (48.0781, 18.0133)
  line L664 (48.0781, 18.0133) -> (48.7641, 15.8014)
  line L665 (48.7641, 15.8014) -> (49.85, 13.8004)
  line L666 (49.85, 13.8004) -> (51.2889, 12.0575)
  line L667 (51.2889, 12.0575) -> (53.0321, 10.6188)
  line L668 (53.0321, 10.6188) -> (55.0331, 9.533)
  line L669 (55.0331, 9.533) -> (57.2447, 8.8467)
  line L670 (57.2447, 8.8467) -> (59.025, 8.6069)
  line L671 (59.025, 8.6069) -> (59.6191, 8.6069)
  line L672 (59.6191, 8.6069) -> (60.2114, 8.6069)
  line L673 (60.2114, 8.6069) -> (61.992, 8.8467)
  line L674 (61.992, 8.8467) -> (64.2038, 9.533)
  line L675 (64.2038, 9.533) -> (66.2048, 10.6188)
  line L676 (66.2048, 10.6188) -> (67.9478, 12.0575)
  line L677 (67.9478, 12.0575) -> (69.3864, 13.8004)
  line L678 (69.3864, 13.8004) -> (70.4723, 15.8014)
  line L679 (70.4723, 15.8014) -> (71.1588, 18.0133)
  line L680 (71.1588, 18.0133) -> (71.3983, 19.7938)
  line L681 (71.3983, 19.7938) -> (71.3983, 20.3861)
  line L682 (71.3983, 20.3861) -> (71.3983, 20.9802)
  line L683 (71.3983, 20.9802) -> (71.1588, 22.7608)
  line L684 (71.1588, 22.7608) -> (70.4723, 24.9711)
  line L685 (70.4723, 24.9711) -> (69.3864, 26.9719)
  line L686 (69.3864, 26.9719) -> (67.9478, 28.7153)
  line L687 (67.9478, 28.7153) -> (66.2048, 30.154)
  line L688 (66.2048, 30.154) -> (64.2038, 31.2398)
  line L689 (64.2038, 31.2398) -> (61.992, 31.9259)
  line L690 (61.992, 31.9259) -> (60.2114, 32.1644)
  line L691 (60.2114, 32.1644) -> (59.6191, 32.1644)
  line L692 (59.6191, 32.1644) -> (59.025, 32.1644)
  line L693 (59.025, 32.1644) -> (57.2447, 31.9259)
  line L694 (57.2447, 31.9259) -> (55.0331, 31.2398)
  line L695 (55.0331, 31.2398) -> (53.0321, 30.154)
  line L696 (53.0321, 30.154) -> (51.2889, 28.7153)
  line L697 (51.2889, 28.7153) -> (49.85, 26.9719)
  line L698 (49.85, 26.9719) -> (48.7641, 24.9711)
  line L699 (48.7641, 24.9711) -> (48.0781, 22.7608)
  line L700 (48.0781, 22.7608) -> (47.8396, 20.9802)
  line L701 (47.8396, 20.9802) -> (47.8396, 20.3861)
  line L702 (96.3383, 12.3757) -> (112.9972, 29.0348)
  line L703 (112.9972, 29.0348) -> (96.3383, 12.3757)
  line L704 (96.3383, 12.3757) -> (96.9269, 12.964)
  line L705 (98.1174, 14.1548) -> (111.8136, 27.8512)
  line L706 (112.4087, 28.4463) -> (112.9972, 29.0348)
  line L707 (112.9974, 12.376) -> (96.3383, 29.0348)
  line L708 (96.3383, 29.0348) -> (112.9972, 12.3757)
  line L709 (112.9972, 12.3757) -> (112.4087, 12.964)
  line L710 (111.2182, 14.1548) -> (97.522, 27.8512)
  line L711 (96.9269, 28.4463) -> (96.3383, 29.0348)
  line L712 (121.9944, 20.5324) -> (121.9944, 19.6516)
  line L713 (121.9944, 19.6516) -> (121.6378, 17.0059)
  line L714 (121.6378, 17.0059) -> (120.618, 13.7207)
  line L715 (120.618, 13.7207) -> (119.0058, 10.7484)
  line L716 (119.0058, 10.7484) -> (116.8682, 8.1588)
  line L717 (116.8682, 8.1588) -> (114.2774, 6.0217)
  line L718 (114.2774, 6.0217) -> (111.3053, 4.4078)
  line L719 (111.3053, 4.4078) -> (108.0213, 3.3882)
  line L720 (108.0213, 3.3882) -> (105.3754, 3.0326)
  line L721 (105.3754, 3.0326) -> (104.495, 3.0326)
  line L722 (104.495, 3.0326) -> (103.6129, 3.0326)
  line L723 (103.6129, 3.0326) -> (100.9672, 3.3882)
  line L724 (100.9672, 3.3882) -> (97.6818, 4.4078)
  line L725 (97.6818, 4.4078) -> (94.7097, 6.0217)
  line L726 (94.7097, 6.0217) -> (92.1202, 8.1588)
  line L727 (92.1202, 8.1588) -> (89.9828, 10.7484)
  line L728 (89.9828, 10.7484) -> (88.3691, 13.7207)
  line L729 (88.3691, 13.7207) -> (87.3493, 17.0059)
  line L730 (87.3493, 17.0059) -> (86.995, 19.6516)
  line L731 (86.995, 19.6516) -> (86.995, 20.5324)
  line L732 (86.995, 20.5324) -> (86.995, 21.4146)
  line L733 (86.995, 21.4146) -> (87.3493, 24.0603)
  line L734 (87.3493, 24.0603) -> (88.3691, 27.3455)
  line L735 (88.3691, 27.3455) -> (89.9828, 30.3178)
  line L736 (89.9828, 30.3178) -> (92.1202, 32.9073)
  line L737 (92.1202, 32.9073) -> (94.7097, 35.0445)
  line L738 (94.7097, 35.0445) -> (97.6818, 36.6579)
  line L739 (97.6818, 36.6579) -> (100.9672, 37.679)
  line L740 (100.9672, 37.679) -> (103.6129, 38.032)
  line L741 (103.6129, 38.032) -> (104.495, 38.032)
  line L742 (104.495, 38.032) -> (105.3754, 38.032)
  line L743 (105.3754, 38.032) -> (108.0213, 37.679)
  line L744 (108.0213, 37.679) -> (111.3053, 36.6579)
  line L745 (111.3053, 36.6579) -> (114.2774, 35.0445)
  line L746 (114.2774, 35.0445) -> (116.8682, 32.9073)
  line L747 (116.8682, 32.9073) -> (119.0058, 30.3178)
  line L748 (119.0058, 30.3178) -> (120.618, 27.3455)
  line L749 (120.618, 27.3455) -> (121.6378, 24.0603)
  line L750 (121.6378, 24.0603) -> (121.9944, 21.4146)
  line L751 (121.9944, 21.4146) -> (121.9944, 20.5324)
  line L752 (96.1659, 12.2035) -> (96.7531, 12.7905)
  line L753 (97.9439, 13.9825) -> (111.6416, 27.6787)
  line L754 (112.2367, 28.2744) -> (112.8237, 28.8614)
  line L755 (69.0227, 22.4108) -> (69.0214, 22.4136)
  line L756 (69.0214, 22.4136) -> (69.0186, 22.4174)
  line L757 (92.8875, 97.1023) -> (92.8875, 96.5105)
  line L758 (92.8875, 96.5105) -> (93.126, 94.7299)
  line L759 (93.126, 94.7299) -> (93.8126, 92.5176)
  line L760 (93.8126, 92.5176) -> (94.8984, 90.5161)
  line L761 (94.8984, 90.5161) -> (96.3368, 88.7736)
  line L762 (96.3368, 88.7736) -> (98.08, 87.3334)
  line L763 (98.08, 87.3334) -> (100.081, 86.2489)
  line L764 (100.081, 86.2489) -> (102.2929, 85.5631)
  line L765 (102.2929, 85.5631) -> (104.0734, 85.3218)
  line L766 (104.0734, 85.3218) -> (104.667, 85.3218)
  line L767 (104.667, 85.3218) -> (105.2598, 85.3218)
  line L768 (105.2598, 85.3218) -> (107.0401, 85.5631)
  line L769 (107.0401, 85.5631) -> (109.2517, 86.2489)
  line L770 (109.2517, 86.2489) -> (111.2527, 87.3334)
  line L771 (111.2527, 87.3334) -> (112.9959, 88.7736)
  line L772 (112.9959, 88.7736) -> (114.4348, 90.5161)
  line L773 (114.4348, 90.5161) -> (115.5207, 92.5176)
  line L774 (115.5207, 92.5176) -> (116.2067, 94.7299)
  line L775 (116.2067, 94.7299) -> (116.4468, 96.5105)
  line L776 (116.4468, 96.5105) -> (116.4468, 97.1023)
  line L777 (116.4468, 97.1023) -> (116.4468, 97.6966)
  line L778 (116.4468, 97.6966) -> (116.2067, 99.4772)
  line L779 (116.2067, 99.4772) -> (115.5207, 101.687)
  line L780 (115.5207, 101.687) -> (114.4348, 103.6885)
  line L781 (114.4348, 103.6885) -> (112.9959, 105.4309)
  line L782 (112.9959, 105.4309) -> (111.2527, 106.8711)
  line L783 (111.2527, 106.8711) -> (109.2517, 107.9557)
  line L784 (109.2517, 107.9557) -> (107.0401, 108.6415)
  line L785 (107.0401, 108.6415) -> (105.2598, 108.8803)
  line L786 (105.2598, 108.8803) -> (104.667, 108.8803)
  line L787 (104.667, 108.8803) -> (104.0734, 108.8803)
  line L788 (104.0734, 108.8803) -> (102.2929, 108.6415)
  line L789 (102.2929, 108.6415) -> (100.081, 107.9557)
  line L790 (100.081, 107.9557) -> (98.08, 106.8711)
  line L791 (98.08, 106.8711) -> (96.3368, 105.4309)
  line L792 (96.3368, 105.4309) -> (94.8984, 103.6885)
  line L793 (94.8984, 103.6885) -> (93.8126, 101.687)
  line L794 (93.8126, 101.687) -> (93.126, 99.4772)
  line L795 (93.126, 99.4772) -> (92.8875, 97.6966)
  line L796 (92.8875, 97.6966) -> (92.8875, 97.1023)
  line L797 (96.7983, 102.4591) -> (96.8288, 102.4109)
  line L798 (96.8192, 102.5582) -> (96.7983, 102.4591)
  line L799 (112.8857, 93.1069) -> (112.8857, 93.4675)
  line L800 (112.8857, 93.4675) -> (112.8857, 93.9451)
  line L801 (112.8857, 93.9451) -> (112.9146, 95.2405)
  line L802 (112.9146, 95.2405) -> (112.9218, 95.3776)
  line L803 (112.9218, 95.3776) -> (112.9075, 95.8704)
  line L804 (152.071, 81.9207) -> (152.071, 81.3263)
  line L805 (152.071, 81.3263) -> (152.3098, 79.5458)
  line L806 (152.3098, 79.5458) -> (152.9956, 77.336)
  line L807 (152.9956, 77.336) -> (154.0802, 75.3345)
  line L808 (154.0802, 75.3345) -> (155.5203, 73.592)
  line L809 (155.5203, 73.592) -> (157.2628, 72.1519)
  line L810 (157.2628, 72.1519) -> (159.2643, 71.0673)
  line L811 (159.2643, 71.0673) -> (161.4741, 70.3789)
  line L812 (161.4741, 70.3789) -> (163.2546, 70.1402)
  line L813 (163.2546, 70.1402) -> (163.849, 70.1402)
  line L814 (163.849, 70.1402) -> (164.4434, 70.1402)
  line L815 (164.4434, 70.1402) -> (166.2214, 70.3789)
  line L816 (166.2214, 70.3789) -> (168.4337, 71.0673)
  line L817 (168.4337, 71.0673) -> (170.4352, 72.1519)
  line L818 (170.4352, 72.1519) -> (172.1777, 73.592)
  line L819 (172.1777, 73.592) -> (173.6178, 75.3345)
  line L820 (173.6178, 75.3345) -> (174.7024, 77.336)
  line L821 (174.7024, 77.336) -> (175.3908, 79.5458)
  line L822 (175.3908, 79.5458) -> (175.6295, 81.3263)
  line L823 (175.6295, 81.3263) -> (175.6295, 81.9207)
  line L824 (175.6295, 81.9207) -> (175.6295, 82.5151)
  line L825 (175.6295, 82.5151) -> (175.3908, 84.2931)
  line L826 (175.3908, 84.2931) -> (174.7024, 86.5054)
  line L827 (174.7024, 86.5054) -> (173.6178, 88.5069)
  line L828 (173.6178, 88.5069) -> (172.1777, 90.2494)
  line L829 (172.1777, 90.2494) -> (170.4352, 91.6895)
  line L830 (170.4352, 91.6895) -> (168.4337, 92.7741)
  line L831 (168.4337, 92.7741) -> (166.2214, 93.4599)
  line L832 (166.2214, 93.4599) -> (164.4434, 93.6987)
  line L833 (164.4434, 93.6987) -> (163.849, 93.6987)
  line L834 (163.849, 93.6987) -> (163.2546, 93.6987)
  line L835 (163.2546, 93.6987) -> (161.4741, 93.4599)
  line L836 (161.4741, 93.4599) -> (159.2643, 92.7741)
  line L837 (159.2643, 92.7741) -> (157.2628, 91.6895)
  line L838 (157.2628, 91.6895) -> (155.5203, 90.2494)
  line L839 (155.5203, 90.2494) -> (154.0802, 88.5069)
  line L840 (154.0802, 88.5069) -> (152.9956, 86.5054)
  line L841 (152.9956, 86.5054) -> (152.3098, 84.2931)
  line L842 (152.3098, 84.2931) -> (152.071, 82.5151)
  line L843 (152.071, 82.5151) -> (152.071, 81.9207)
  line L844 (188.5683, 39.4519) -> (188.5683, 38.8601)
  line L845 (188.5683, 38.8601) -> (188.807, 37.0795)
  line L846 (188.807, 37.0795) -> (189.4928, 34.868)
  line L847 (189.4928, 34.868) -> (190.5774, 32.8672)
  line L848 (190.5774, 32.8672) -> (192.0176, 31.124)
  line L849 (192.0176, 31.124) -> (193.76, 29.6853)
  line L850 (193.76, 29.6853) -> (195.7616, 28.5995)
  line L851 (195.7616, 28.5995) -> (197.9714, 27.9129)
  line L852 (197.9714, 27.9129) -> (199.7519, 27.6734)
  line L853 (199.7519, 27.6734) -> (200.3463, 27.6734)
  line L854 (200.3463, 27.6734) -> (200.9406, 27.6734)
  line L855 (200.9406, 27.6734) -> (202.7186, 27.9129)
  line L856 (202.7186, 27.9129) -> (204.931, 28.5995)
  line L857 (204.931, 28.5995) -> (206.9325, 29.6853)
  line L858 (206.9325, 29.6853) -> (208.6749, 31.124)
  line L859 (208.6749, 31.124) -> (210.1151, 32.8672)
  line L860 (210.1151, 32.8672) -> (211.1997, 34.868)
  line L861 (211.1997, 34.868) -> (211.888, 37.0795)
  line L862 (211.888, 37.0795) -> (212.1268, 38.8601)
  line L863 (212.1268, 38.8601) -> (212.1268, 39.4519)
  line L864 (212.1268, 39.4519) -> (212.1268, 40.0463)
  line L865 (212.1268, 40.0463) -> (211.888, 41.8268)
  line L866 (211.888, 41.8268) -> (211.1997, 44.0391)
  line L867 (211.1997, 44.0391) -> (210.1151, 46.0407)
  line L868 (210.1151, 46.0407) -> (208.6749, 47.7831)
  line L869 (208.6749, 47.7831) -> (206.9325, 49.2207)
  line L870 (206.9325, 49.2207) -> (204.931, 50.3079)
  line L871 (204.931, 50.3079) -> (202.7186, 50.9937)
  line L872 (202.7186, 50.9937) -> (200.9406, 51.2324)
  line L873 (200.9406, 51.2324) -> (200.3463, 51.2324)
  line L874 (200.3463, 51.2324) -> (199.7519, 51.2324)
  line L875 (199.7519, 51.2324) -> (197.9714, 50.9937)
  line L876 (197.9714, 50.9937) -> (195.7616, 50.3079)
  line L877 (195.7616, 50.3079) -> (193.76, 49.2207)
  line L878 (193.76, 49.2207) -> (192.0176, 47.7831)
  line L879 (192.0176, 47.7831) -> (190.5774, 46.0407)
  line L880 (190.5774, 46.0407) -> (189.4928, 44.0391)
  line L881 (189.4928, 44.0391) -> (188.807, 41.8268)
  line L882 (188.807, 41.8268) -> (188.5683, 40.0463)
  line L883 (188.5683, 40.0463) -> (188.5683, 39.4519)
  line L884 (33.6664, 82.0883) -> (33.6664, 81.4965)
  line L885 (33.6664, 81.4965) -> (33.9049, 79.716)
  line L886 (33.9049, 79.716) -> (34.5909, 77.5036)
  line L887 (34.5909, 77.5036) -> (35.6771, 75.5047)
  line L888 (35.6771, 75.5047) -> (37.1157, 73.7597)
  line L889 (37.1157, 73.7597) -> (38.8589, 72.322)
  line L890 (38.8589, 72.322) -> (40.8599, 71.2349)
  line L891 (40.8599, 71.2349) -> (43.0718, 70.5491)
  line L892 (43.0718, 70.5491) -> (44.8518, 70.3104)
  line L893 (44.8518, 70.3104) -> (45.4459, 70.3104)
  line L894 (45.4459, 70.3104) -> (46.0385, 70.3104)
  line L895 (46.0385, 70.3104) -> (47.819, 70.5491)
  line L896 (47.819, 70.5491) -> (50.0306, 71.2349)
  line L897 (50.0306, 71.2349) -> (52.0301, 72.322)
  line L898 (52.0301, 72.322) -> (53.7733, 73.7597)
  line L899 (53.7733, 73.7597) -> (55.2122, 75.5047)
  line L900 (55.2122, 75.5047) -> (56.298, 77.5036)
  line L901 (56.298, 77.5036) -> (56.9843, 79.716)
  line L902 (56.9843, 79.716) -> (57.2241, 81.4965)
  line L903 (57.2241, 81.4965) -> (57.2241, 82.0883)
  line L904 (57.2241, 82.0883) -> (57.2241, 82.6827)
  line L905 (57.2241, 82.6827) -> (56.9843, 84.4632)
  line L906 (56.9843, 84.4632) -> (56.298, 86.6756)
  line L907 (56.298, 86.6756) -> (55.2122, 88.6771)
  line L908 (55.2122, 88.6771) -> (53.7733, 90.4195)
  line L909 (53.7733, 90.4195) -> (52.0301, 91.8572)
  line L910 (52.0301, 91.8572) -> (50.0306, 92.9443)
  line L911 (50.0306, 92.9443) -> (47.819, 93.6301)
  line L912 (47.819, 93.6301) -> (46.0385, 93.8689)
  line L913 (46.0385, 93.8689) -> (45.4459, 93.8689)
  line L914 (45.4459, 93.8689) -> (44.8518, 93.8689)
  line L915 (44.8518, 93.8689) -> (43.0718, 93.6301)
  line L916 (43.0718, 93.6301) -> (40.8599, 92.9443)
  line L917 (40.8599, 92.9443) -> (38.8589, 91.8572)
  line L918 (38.8589, 91.8572) -> (37.1157, 90.4195)
  line L919 (37.1157, 90.4195) -> (35.6771, 88.6771)
  line L920 (35.6771, 88.6771) -> (34.5909, 86.6756)
  line L921 (34.5909, 86.6756) -> (33.9049, 84.4632)
  line L922 (33.9049, 84.4632) -> (33.6664, 82.6827)
  line L923 (33.6664, 82.6827) -> (33.6664, 82.0883)
  line L924 (-2.6711, 39.396) -> (-2.6711, 38.8042)
  line L925 (-2.6711, 38.8042) -> (-2.4326, 37.0237)
  line L926 (-2.4326, 37.0237) -> (-1.7463, 34.8116)